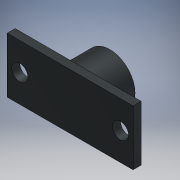
# Autodesk Inventor part: 磁鐵b
Saved by Autodesk Inventor 2017 (Build 210142000, 142)
## iProperties
Part Number: 磁鐵b
Material: SS41
Document SubType Name: Modeling
Designer: G
Density: 7.85 g/cm^3
Appearance: 鐵灰色
Author: G
Autodesk Inventor part; units mm, degrees
ref_plane "YZ Plane" through (0, 0, 0) normal (1, 0, 0) x (0, 1, 0)
ref_plane "XZ Plane" through (0, 0, 0) normal (0, 1, 0) x (-1, 0, 0)
ref_plane "XY Plane" through (0, 0, 0) normal (0, 0, 1) x (1, 0, 0)
sketch "草圖1" plane through (0, 0, 0) normal (0, 0, 1) x (1, 0, 0)
  line L0 (0, 7.9) -> (5, 7.9)
  line L1 (5, 7.9) -> (5, 1.6)
  line L2 (5, 1.6) -> (15, 1.6)
  line L3 (15, 1.6) -> (15, 0)
  line L4 (15, 0) -> (0, 0)
  line L5 (0, 7.9) -> (0, 0)
  point P0 (0, 0)
  dimension "d1" = 1.6
  dimension "d2" = 10
  dimension "d3" = 30
  dimension "d4" = 6.3
  constraints: 12 end point, 4 perpendicular, 1 coincident, 1 horizontal, 1 vertical
  measures "d1" distance of L2.end L3.end
  measures "d2" diameter of L1 L5
  measures "d3" diameter of L3 L5
  measures "d4" distance of L0.end L1.end
revolve "迴轉1" add sketch "草圖1" angle 360 about axis through (0, 7.9, 0) along (0, -1, 0)
sketch "草圖2" plane through (0, 0, 0) normal (0, 1, 0) x (-1, 0, 0)
  line L0 (12.5, -5.5) -> (-12.5, -5.5)
  line L1 (-12.5, -5.5) -> (-12.5, 5.5)
  line L2 (-12.5, 5.5) -> (12.5, 5.5)
  line L3 (12.5, 5.5) -> (12.5, -5.5)
  circle A0 centre (10, 0) radius 1.6
  circle A1 centre (-10, 0) radius 1.6
  line L4 (10, 0) -> (-10, 0) construction
  point P0 (0, 0)
  point P1 (0, -5.5)
  point P2 (-12.5, 0)
  point P3 (0, 0)
  dimension "d6" = 11
  dimension "d7" = 25
  dimension "d8" = 3.2
  dimension "d9" = 20
  constraints: 10 end point, 3 horizontal alignment, 3 midpoint, 2 centre point, 2 horizontal, 2 parallel, 1 coincident, 1 equal radius, 1 perpendicular, 1 vertical alignment
  measures "d6" distance of L0.end L1.end
  measures "d7" distance of L0.start L0.end
  measures "d8" diameter of A0
  measures "d9" distance of L4.end L4.start
extrude "擠出1" cut sketch "草圖2" along normal through all keep common part
